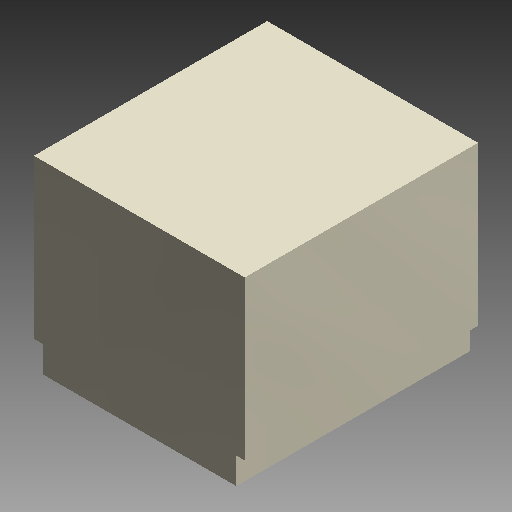
# Autodesk Inventor part: C-GRID-02-70543
Saved by Autodesk Inventor 2018.2 (Build 222227000, 227)
## iProperties
Part Number: C-GRID-02-70543
Material: Generic
Document SubType Name: Modeling
Designer: autocad
Appearance: 70543-02, C-GRID-02-70543
Author: autocad
Autodesk Inventor part; units mm, degrees
ref_plane "YZ Plane" through (0, 0, 0) normal (1, 0, 0) x (0, 1, 0)
ref_plane "XZ Plane" through (0, 0, 0) normal (0, 1, 0) x (-1, 0, 0)
ref_plane "XY Plane" through (0, 0, 0) normal (0, 0, 1) x (1, 0, 0)
sketch "70543-02, C-GRID-02-70543_91" plane through (0, 0, 0) normal (0, 0, 1) x (1, 0, 0)
  line L0 (3.8095, 2.8697) -> (3.8095, -2.857)
  line L1 (3.8095, -2.857) -> (3.5047, -2.857)
  line L2 (3.5047, -2.857) -> (3.5047, -3.8095)
  line L3 (3.5047, -3.8095) -> (-3.492, -3.8095)
  line L4 (-3.492, -3.8095) -> (-3.492, -2.857)
  line L5 (-3.492, -2.857) -> (-3.8095, -2.857)
  line L6 (-3.8095, -2.857) -> (-3.8095, 2.8697)
  line L7 (-3.8095, 2.8697) -> (3.8095, 2.8697)
  constraints: 16 end point
extrude "Extrusion1" add sketch "70543-02, C-GRID-02-70543_91" along normal blind 8.43
body "Solid1"
